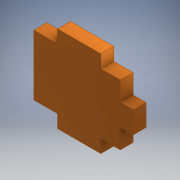
# Autodesk Inventor part: Top
Saved by Autodesk Inventor 2018 (Build 220112000, 112)
## iProperties
Created: 2020-03-13
Part Number: Top
Material: Oro
Document SubType Name: Modeling
Designer: joser
Density: 19.3 g/cm^3
Appearance: Metal 1600F
Author: joser
Autodesk Inventor part; units mm, degrees
ref_plane "YZ Plane" through (0, 0, 0) normal (1, 0, 0) x (0, 1, 0)
ref_plane "XZ Plane" through (0, 0, 0) normal (0, 1, 0) x (-1, 0, 0)
ref_plane "XY Plane" through (0, 0, 0) normal (0, 0, 1) x (1, 0, 0)
sketch "Boceto1" plane through (0, 0, 0) normal (0, 1, 0) x (-1, 0, 0)
  line L0 (17.5, 7.5) -> (7.5, 7.5)
  line L1 (0, 0) -> (0, -5)
  line L2 (7.5, -12.5) -> (17.5, -12.5)
  line L3 (23, -9.5) -> (23, 4.5)
  line L4 (17.5, 4.5) -> (17.5, 7.5)
  line L5 (7.5, 4.5) -> (7.5, 7.5)
  line L6 (3, 4.5) -> (7.5, 4.5)
  line L7 (17.5, 4.5) -> (23, 4.5)
  line L8 (17.5, -9.5) -> (17.5, -12.5)
  line L9 (7.5, -9.5) -> (7.5, -12.5)
  line L10 (23, -9.5) -> (17.5, -9.5)
  line L11 (7.5, -9.5) -> (3, -9.5)
  line L12 (3, -5) -> (0, -5)
  line L13 (3, 0) -> (0, 0)
  line L14 (3, -9.5) -> (3, -5)
  line L15 (3, 0) -> (3, 4.5)
  point P0 (0, -2.5)
  point P1 (12.5, -12.5)
  dimension "d0" = 23
  dimension "d1" = 20
  dimension "d2" = 10
  dimension "d3" = 5
  dimension "d4" = 3
  dimension "d5" = 3
  dimension "d11" = 7.5
  constraints: 32 end point, 7 equal length, 7 parallel, 6 perpendicular, 4 horizontal, 2 coincident, 2 midpoint
  measures "d0" distance between parallel lines of L1 L3
  measures "d1" distance between parallel lines of L2 L0
  measures "d2" distance between parallel lines of L5 L4
  measures "d3" distance between parallel lines of L12 L13
  measures "d4" distance between parallel lines of L10 L2
  measures "d5" distance between parallel lines of L15 L1
  measures "d11" distance between parallel lines of L1 L5
extrude "Extrusión1" add sketch "Boceto1" along normal blind 3
